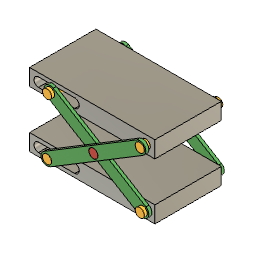
Weekend Project_1 v2 (Autodesk Fusion 360 design; units mm, degrees)
Autodesk Fusion 360 part; units mm, degrees
sketch "Sketch1" plane through (0, 0, 0) normal (0, 1, 0) x (1, 0, 0)
  line L0 (83, -11) -> (-83, -11)
  line L1 (-83, -11) -> (-83, 11)
  line L2 (-83, 11) -> (83, 11)
  line L3 (83, 11) -> (83, -11)
  line L4 (83, -11) -> (-83, 11) construction
  line L5 (-83, -11) -> (83, 11) construction
  line L6 (-71, -6) -> (-23, -6)
  arc A0 (-23, -6) -> (-23, 6) centre (-23, 0) ccw
  line L7 (-23, 6) -> (-71, 6)
  arc A1 (-71, 6) -> (-71, -6) centre (-71, 0) ccw
  line L8 (-71, 0) -> (-23, 0) construction
  circle A2 centre (71, 0) radius 6
  circle A3 centre (-71, 0) radius 6
  dimension "d1" = 166
  dimension "d2" = 22
  dimension "d3" = 12
  dimension "d4" = 12
  dimension "d5" = 6
  dimension "d6" = 12
  dimension "d7" = 48
  constraint horizontal L0
  constraint perpendicular L0 L1
  constraint parallel L0 L2
  constraint parallel L1 L3
  constraint coincident L4 origin
  constraint coincident L5 origin
  constraint tangent L6 A0
  constraint tangent A0 L7
  constraint parallel L6 L7
  constraint tangent L7 A1
  constraint tangent L6 A1
  constraint horizontal L8
  constraint concentric A1 A3
  constraint coincident L6.start A3
  measures "d1" distance of L1.end L2.end
  measures "d2" distance of L0.start L2.end
  measures "d3" diameter of A2
  measures "d4" distance of L3 A2.centre
  measures "d5" radius of A1
  measures "d6" distance of L1 A1.centre
  measures "d7" distance of A1.centre A0.centre
extrude "Extrude1" add sketch "Sketch1" along normal mid plane 88 makes body 1 in component "base"
extrude "Extrude1'" add sketch "Sketch1" along normal mid plane 104 separate body contours A2 makes body 2 in component "pin"
extrude "Extrude1''" add sketch "Sketch1" along normal mid plane 104 separate body contours A1 A3 makes body 3 in component "Component"
sketch "Sketch2" plane through (0, -44, 0) normal (0, -1, 0) x (1, 0, 0)
  circle A0 centre (71, 0) radius 6
  line L0 (-23, -6) -> (-71, -6)
  arc A1 (-71, 6) -> (-71, -6) centre (-71, 0) ccw
  line L1 (-71, 6) -> (-23, 6)
  arc A2 (-23, -6) -> (-23, 6) centre (-23, 0) ccw
  line L2 (-83, -11) -> (83, -11)
  line L3 (83, -11) -> (83, 11)
  line L4 (83, 11) -> (-83, 11)
  line L5 (-83, 11) -> (-83, -11)
  line L6 (-72.2248, 14.0943) -> (69.7752, -7.9057)
  arc A3 (69.7752, -7.9057) -> (72.2248, 7.9057) centre (71, 0) ccw
  line L7 (72.2248, 7.9057) -> (-69.7752, 29.9057)
  arc A4 (-69.7752, 29.9057) -> (-72.2248, 14.0943) centre (-71, 22) ccw
  line L8 (-71, 22) -> (71, 0) construction
  circle A5 centre (71, 0) radius 6
  circle A6 centre (-71, 22) radius 6
  circle A7 centre (0, 11) radius 6
  dimension "d35" = 8
  constraint tangent L6 A3
  constraint tangent A3 L7
  constraint parallel L6 L7
  constraint tangent L7 A4
  constraint tangent L6 A4
  constraint coincident A0.centre A3.centre
  constraint coincident A4.centre L8.start
  constraint midpoint L4 A7.centre
  constraint equal A6 A7
  measures "d35" radius of A3
extrude "Extrude1'''" add sketch "Sketch2" along normal blind 4 separate body contours L4 L6 L7 A4 A7 | L4 L6 A3 L7 A7 makes body 4 in component "scissor"
extrude "Extrude1''''" add sketch "Sketch2" along normal blind 8 separate body contours L4 A7 | L4 A7 makes body 5 in component "rivet"
component "base" placed x (1, 0, 0) y (0, 1, 0) z (0, 0, 1) at (0, 0, 0)
component "pin" placed x (1, 0, 0) y (0, 1, 0) z (0, 0, 1) at (0, 0, 0)
component "Component" placed x (-0.647278, 0, -0.762254) y (0, 1, 0) z (0.762254, 0, -0.647278) at (-68.9567, 0, -54.1201)
component "Component" placed x (0.762254, 0, -0.647278) y (0, 1, 0) z (0.647278, 0, 0.762254) at (31.1201, 0, 62.7263)
component "pin" placed x (0, 0, -1) y (0, 1, 0) z (1, 0, 0) at (71, 0, 179.683)
component "base" placed x (1, 0, 0) y (0, 1, 0) z (0, 0, 1) at (0, 0, 108.683)
component "scissor" placed x (-0.762254, 0, 0.647278) y (0, 1, 0) z (-0.647278, 0, -0.762254) at (31.1201, 0, 62.7263)
component "rivet" placed x (0.922383, 0, -0.386278) y (0, 1, 0) z (0.386278, 0, 0.922383) at (19.7509, 0, 44.1953)
component "scissor" placed x (0.530655, 0, 0.847588) y (0, 1, 0) z (-0.847588, 0, 0.530655) at (33.3235, -4, 48.5043)
component "scissor" placed x (0.530655, 0, 0.847588) y (0, 1, 0) z (-0.847588, 0, 0.530655) at (33.3235, 92, 48.5043)
component "scissor" placed x (-0.762254, 0, 0.647278) y (0, 1, 0) z (-0.647278, 0, -0.762254) at (31.1201, 96, 62.7263)
component "rivet" placed x (-0.762254, 0, -0.647278) y (0, 1, 0) z (0.647278, 0, -0.762254) at (16.8799, 96, 62.7263)
